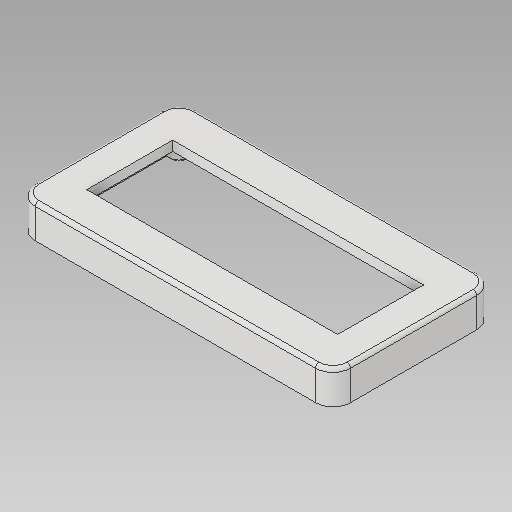
# Autodesk Inventor part: PANTALLA BASE
Saved by Autodesk Inventor 2019 (Build 230136000, 136)
## iProperties
Created: 2019-08-04
Part Number: PANTALLA BASE
Material: Plástico ABS
Document SubType Name: Modeling
Designer: Luis Pujol
Density: 1.06 g/cm^3
Appearance: Suave - Blanco
Author: Luis Pujol
## iProperties of the stored document PANTALLA BASE_3DPrint.ipt
Created: 2019-08-04
Part Number: PANTALLA BASE_3DPrint
Material: Genérico
Document SubType Name: Modeling
Designer: Luis Pujol
Density: 1 g/cm^3
Appearance: Valor por defecto
Author: Luis Pujol
Autodesk Inventor part; units mm, degrees
ref_plane "YZ Plane" through (0, 0, 0) normal (1, 0, 0) x (0, 1, 0)
ref_plane "XZ Plane" through (0, 0, 0) normal (0, 1, 0) x (-1, 0, 0)
ref_plane "XY Plane" through (0, 0, 0) normal (0, 0, 1) x (1, 0, 0)
sketch "Boceto1" plane through (0, 0, 0) normal (0, 1, 0) x (-1, 0, 0)
  line L0 (45, 23) -> (-45, 23)
  line L1 (-45, 23) -> (-45, -23)
  line L2 (-45, -23) -> (45, -23)
  line L3 (45, -23) -> (45, 23)
  line L4 (45, 23) -> (-45, -23) construction
  line L5 (-45, 23) -> (45, -23) construction
  point P0 (0, 0)
  dimension "d0" = 90
  dimension "d1" = 46
  constraints: 12 end point, 2 midpoint, 2 parallel, 1 horizontal, 1 perpendicular
  measures "d0" distance of L2.end L1.end
  measures "d1" distance of L1.end L0.end
extrude "Extrusión1" add sketch "Boceto1" along normal blind 9.5
fillet "Empalme1" radius 5 4 edges at (45, 4.75, 23) (45, 4.75, -23) (-45, 4.75, 23) (-45, 4.75, -23)
shell "Vaciado1" thickness 2.8 removed faces 1 at (-13.3333, 0, -7.6667)
fillet "Empalme2" radius 1 8 edges at (43.5355, 9.5, 21.5355) (45, 9.5, 0) (43.5355, 9.5, -21.5355) (0, 9.5, -23) (-43.5355, 9.5, -21.5355) (-45, 9.5, 0) (-43.5355, 9.5, 21.5355) (0, 9.5, 23)
sketch "Boceto2" plane through (0, 9.5, 0) normal (0, 1, 0) x (1, 0, 0)
  line L0 (-35.8, -12.5) -> (35.8, -12.5)
  line L1 (35.8, -12.5) -> (35.8, 12)
  line L2 (35.8, 12) -> (-35.8, 12)
  line L3 (-35.8, 12) -> (-35.8, -12.5)
  line L4 (40, 23) -> (-40, 23) projected
  line L5 (-40, -23) -> (40, -23) projected
  point P0 (0, 0)
  point P1 (0, 12)
  dimension "d7" = 11
  dimension "d10" = 24.5
  dimension "d11" = 71.6
  constraints: 8 end point, 2 parallel, 1 horizontal, 1 midpoint, 1 perpendicular, 1 vertical alignment
  measures "d7" distance between parallel lines of L4 L2
  measures "d10" distance of L2.end L0.start
  measures "d11" distance of L1.end L2.end
extrude "Extrusión2" cut sketch "Boceto2" against normal blind 9.5
sketch "Boceto3" plane through (-40, 6.7, -20.2) normal (0, -1, 0) x (1, 0, 0)
  line L0 (75.8, 32.7) -> (75.8, 8.2) projected
  line L1 (75.8, 8.2) -> (4.2, 8.2) projected
  line L2 (4.2, 8.2) -> (4.2, 32.7) projected
  line L3 (4.2, 32.7) -> (75.8, 32.7) projected
  arc A0 (-2.2, 2.2) -> (0, 0) centre (0, 2.2) ccw projected
  line L4 (80, 0) -> (0, 0) projected
  arc A1 (80, 0) -> (82.2, 2.2) centre (80, 2.2) ccw projected
  line L5 (82.2, 38.2) -> (82.2, 2.2) projected
  arc A2 (82.2, 38.2) -> (80, 40.4) centre (80, 38.2) ccw projected
  line L6 (0, 40.4) -> (80, 40.4) projected
  arc A3 (0, 40.4) -> (-2.2, 38.2) centre (0, 38.2) ccw projected
  line L7 (-2.2, 2.2) -> (-2.2, 38.2) projected
  line L8 (80, -2.8) -> (0, -2.8) construction
  line L9 (66.1552, -2.8) -> (66.1552, 20.2) construction
  line L10 (0, 43.2) -> (80, 43.2) construction
  line L11 (77.5, 35.7) -> (2.5, 35.7) construction
  line L12 (2.5, 35.7) -> (2.5, 4.7) construction
  line L13 (2.5, 4.7) -> (77.5, 4.7) construction
  line L14 (77.5, 4.7) -> (77.5, 35.7) construction
  line L15 (77.5, 35.7) -> (2.5, 4.7) construction
  line L16 (2.5, 35.7) -> (77.5, 4.7) construction
  circle A4 centre (77.5, 4.7) radius 2.75
  circle A5 centre (2.5, 4.7) radius 2.75
  circle A6 centre (2.5, 35.7) radius 2.75
  circle A7 centre (77.5, 35.7) radius 2.75
  point P0 (40, 20.2)
  dimension "d14" = 23
  dimension "d15" = 75
  dimension "d16" = 31
  dimension "d17" = 5.5
  dimension "d18" = 5.5
  dimension "d19" = 5.5
  dimension "d20" = 5.5
  constraints: 14 end point, 4 centre point, 4 coincident, 2 midpoint, 2 parallel, 2 perpendicular, 1 horizontal, 1 point on line
  measures "d14" distance of L9.start L9.end
  measures "d15" distance of L13.end L12.end
  measures "d16" distance of L12.end L11.end
  measures "d17" diameter of A4
  measures "d18" diameter of A5
  measures "d19" diameter of A6
  measures "d20" diameter of A7
extrude "Extrusión3" add sketch "Boceto3" along normal blind 3.3 contours A4 | A5 | A6 | A7
fillet "Empalme3" radius 0.5 8 edges at (34.75, 6.7, -15.5) (34.75, 3.4, -15.5) (34.75, 3.4, 15.5) (34.75, 6.7, 15.5) (-40.25, 3.4, -15.5) (-40.25, 6.7, -15.5) (-40.25, 3.4, 15.5) (-40.25, 6.7, 15.5)
sketch "Boceto4" plane through (37.5, 3.4, 15.5) normal (0, -1, 0) x (1, 0, 0)
  circle A0 centre (0, -31) radius 2.25 projected
  circle A1 centre (-75, -31) radius 2.25 projected
  circle A2 centre (-75, 0) radius 2.25 projected
  circle A3 centre (0, 0) radius 2.25 projected
  point P0 (-37.5, -15.5)
hole "Agujero1" at (37.5, 3.4, -15.5) at (-37.5, 3.4, -15.5) at (-37.5, 3.4, 15.5) at (37.5, 3.4, 15.5) direction (0, 1, 0) diameter 1.8 depth 4 tip angle 118 countersink diameter 2.5 countersink angle 90
